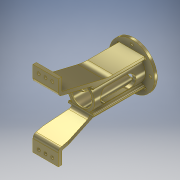
# Autodesk Inventor part: reverse gear standard 101
Saved by Autodesk Inventor 2017 (Build 210142000, 142)
## iProperties
Created: 2018-11-13
Part Number: reverse gear standard 101
Material: Generic
Document SubType Name: Modeling
Designer: User
Density: 1 g/cm^3
Appearance: Default
Author: User
Autodesk Inventor part; units mm, degrees
sketch "Sketch1" plane through (0, 0, 0) normal (0, 1, 0) x (-1, 0, 0)
  circle A0 centre (0, 0) radius 27
  circle A1 centre (0, 0) radius 14
  circle A2 centre (0, 0) radius 16
  circle A3 centre (0, 0) radius 12
  circle A4 centre (0, 0) radius 22 construction
  circle A5 centre (0, -22) radius 1.75
  circle A6 centre (15.5563, -15.5563) radius 1.75
  circle A7 centre (22, 0) radius 1.75
  circle A8 centre (15.5563, 15.5563) radius 1.75
  circle A9 centre (0, 22) radius 1.75
  circle A10 centre (-15.5563, 15.5563) radius 1.75
  circle A11 centre (-22, 0) radius 1.75
  circle A12 centre (-15.5563, -15.5563) radius 1.75
  dimension "d6" = 44
  dimension "d2" = 54
  dimension "d3" = 28
  dimension "d4" = 32
  dimension "d5" = 24
  dimension "d7" = 3.5
  dimension "d8" = 360
  dimension "d9" = 15.5564
  constraints: 12 centre point, 5 coincident, 1 vertical alignment, 19 other
  measures "d2" diameter of A0
  measures "d3" diameter of A1
  measures "d4" diameter of A2
  measures "d5" diameter of A3
  measures "d7" diameter of A5
  measures "d9" horizontal distance of A0.centre A6.centre
extrude "Extrusion1" add sketch "Sketch1" along normal blind 3 contours A0
extrude "Extrusion3" add sketch "Sketch1" against normal blind 60 contours A1 | A2
extrude "Extrusion4" cut sketch "Sketch1" against normal blind 1 contours A1
ref_plane "Work Plane1" through (0, 0, 0) normal (0, 0, 1) x (1, 0, 0)
ref_plane "Work Plane2" through (0, 0, 0) normal (1, 0, 0) x (0, 1, 0)
sketch "Sketch4" plane through (0, 0, 0) normal (1, 0, 0) x (0, 1, 0)
  line L0 (-102, -45) -> (-102, -30.9493)
  line L1 (-98.1581, -26.0853) -> (-63.8419, -17.9147)
  line L2 (-60, -12) -> (-60, 12)
  line L3 (-60, -13.0507) -> (-60, -12)
  line L4 (0, 27) -> (0, -27)
  line L5 (-60, -12) -> (0, -12)
  line L6 (-1, -12) -> (-60, -12)
  line L7 (0, -12) -> (0, -17)
  line L8 (0, -17) -> (-37.1036, -17)
  line L9 (-96.4652, -29.788) -> (-48.7347, -18.3716)
  line L10 (-102, -45) -> (-98, -45)
  line L11 (-98, -45) -> (-98, -31.7331)
  arc A0 (-96.4652, -29.788) -> (-98, -31.7331) centre (-96, -31.7331) ccw
  arc A1 (-98.1581, -26.0853) -> (-102, -30.9493) centre (-97, -30.9493) ccw
  arc A2 (-63.8419, -17.9147) -> (-60, -13.0507) centre (-65, -13.0507) ccw
  arc A3 (-37.1036, -17) -> (-48.7347, -18.3716) centre (-37.1036, -67) ccw
  point P0 (0, 0)
  point P1 (0, 0)
  point P2 (-102, -27)
  point P3 (0, 27)
  point P4 (0, -27)
  point P5 (-43, -17)
  point P6 (-3, -16)
  point P7 (-60, -16)
  dimension "d20" = 18
  dimension "d21" = 43
  dimension "d22" = 4
  dimension "d23" = 2
  dimension "d24" = 5
  dimension "d25" = 50
  dimension "d26" = 13.451
  dimension "d27" = 166.608
  dimension "d28" = 33
  dimension "d29" = 5
  dimension "d30" = 38
  constraints: 22 end point, 8 point on circle, 8 tangent, 5 point on line, 4 centre point, 2 perpendicular, 2 vertical, 1 equal radius, 1 horizontal, 5 other
  measures "d20" distance of L0.start point (-102, -27)
  measures "d21" distance of L7.end point (-43, -17)
  measures "d22" distance of L0.start L10.end
  measures "d23" radius of A0
  measures "d24" radius of A1
  measures "d25" radius of A3
  measures "d26" angle of L6 L9
  measures "d27" angle of L6 L1
  measures "d28" distance between parallel lines of L6 L10
  measures "d29" distance between parallel lines of L6 L8
  measures "d30" distance between parallel lines of L2 L11
extrude "Extrusion5" add sketch "Sketch4" along normal mid plane 30
ref_plane "Work Plane8" through (0, 0, -55) normal (0, 0, 1) x (1, 0, 0)
sketch "Sketch9" plane through (0, 0, -55) normal (0, 0, 1) x (1, 0, 0)
  line L0 (-15, 0) -> (-14.5672, 0) projected
  line L1 (14.5672, 0) -> (-14.5672, 0) projected
  line L2 (14.5672, 0) -> (15, 0) projected
  line L3 (15, -37.1036) -> (15, 0) projected
  line L4 (-15, -37.1036) -> (15, -37.1036) projected
  line L5 (-15, 0) -> (-15, -37.1036) projected
  line L6 (-15, -48.7347) -> (15, -48.7347) projected
  line L7 (15, -96.4652) -> (15, -48.7347) projected
  line L8 (-15, -96.4652) -> (15, -96.4652) projected
  line L9 (-15, -48.7347) -> (-15, -96.4652) projected
  line L10 (-15, -48.7347) -> (-15, -37.1036) projected
  line L11 (15, -37.1036) -> (15, -48.7347) projected
  line L12 (15, 0) -> (15, -60) projected
  line L13 (12, -1) -> (-12, -1) projected
  line L14 (14.5672, 0) -> (15, 0) projected
  line L15 (15, 0) -> (8, 0)
  line L16 (-14, 0) -> (14, 0) projected
  line L17 (-15, 0) -> (-15, -37.1036) projected
  line L18 (-15, 0) -> (-8, 0)
  line L19 (15, 0) -> (15, -89.9)
  line L20 (-15, 0) -> (-15, -89.9)
  line L21 (8, 0) -> (8, -44.2)
  line L22 (-8, 0) -> (-8, -44.2)
  line L23 (8, -44.2) -> (15, -89.9)
  line L24 (-8, -44.2) -> (-15, -89.9)
  point P0 (0, 0)
  point P1 (0, -1)
  point P2 (7.2111, 0)
  point P3 (-7.2111, 0)
  dimension "d85" = 7
  dimension "d86" = 7
  dimension "d87" = 89.9
  dimension "d88" = 89.9
  dimension "d89" = 44.2
  dimension "d90" = 44.2
  constraints: 16 end point, 4 point on line, 2 vertical
  measures "d85" distance of L2.end L15.end
  measures "d86" distance of L0.start L18.end
  measures "d87" distance of L2.end L19.end
  measures "d88" distance of L0.start L20.end
  measures "d89" distance of L15.end L21.end
  measures "d90" distance of L18.end L22.end
extrude "Extrusion7" cut sketch "Sketch9" along normal blind 40 contours L0 L1 L22 L4 L5 | L4 L22 L24 L6 L10 | L6 L24 L9 | L21 L1 L2 L3 L4 | L4 L11 L6 L23 L21 | L6 L7 L23
sketch "Sketch10" plane through (-15, -98, -31.7331) normal (0, 1, 0) x (1, 0, 0)
  line L0 (30, 13.2669) -> (0, 13.2669)
  circle A0 centre (7, 7.2669) radius 1.75
  circle A1 centre (15, 7.2669) radius 1.75
  circle A2 centre (23, 7.2669) radius 1.75
  point P0 (15, -31.7331)
  point P1 (15, -31.7331)
  dimension "d95" = 3.5
  dimension "d96" = 3.5
  dimension "d97" = 6
  dimension "d98" = 6
  dimension "d99" = 6
  dimension "d100" = 9.2195
  dimension "d101" = 16.1555
  dimension "d102" = 23.7697
  dimension "d103" = 45
  dimension "d104" = 45
  dimension "d105" = 47.4342
  dimension "d106" = 0
  dimension "d107" = 47.4342
  constraints: 3 centre point, 2 end point, 1 equal radius, 1 horizontal
  measures "d95" diameter of A0
  measures "d96" diameter of A1
  measures "d97" distance from line of A2.centre L0
  measures "d98" distance from line of A1.centre L0
  measures "d99" distance from line of A0.centre L0
  measures "d100" distance of L0.start A2.centre
  measures "d101" distance of L0.start A1.centre
  measures "d102" distance of L0.start A0.centre
  measures "d103" distance from line of point (15, -31.733) L0
  measures "d104" distance from line of point (15, -31.733) L0
  measures "d105" distance of point (15, -31.733) L0.start
  measures "d106" distance of point (15, -31.733) point (15, -31.733)
  measures "d107" distance of point (15, -31.733) L0.end
extrude "Extrusion8" cut sketch "Sketch10" against normal through all
mirror "Mirror1" about plane through (0, 0, 0) normal (0, 0, 1) of "Extrusion5"
mirror "Mirror2" about plane through (0, 0, 0) normal (0, 0, 1) of "Extrusion8"
fillet "Fillet1" radius 1 1 edges at (12, -60, 0)
ref_plane "Work Plane9" through (34, 0, 0) normal (1, 0, 0) x (0, 1, 0)
sketch "Sketch12" plane through (34, 0, 0) normal (1, 0, 0) x (0, 1, 0)
  arc A0 (-45, 8) -> (-45, -8) centre (-45, 0) ccw
  line L0 (-45, -8) -> (-19, -8)
  arc A1 (-19, -8) -> (-19, 8) centre (-19, 0) ccw
  line L1 (-19, 8) -> (-45, 8)
  point P0 (0, 0)
  point P1 (0, 0)
  dimension "d113" = 16
  dimension "d114" = 26
  dimension "d115" = 8
  dimension "d116" = 8
  dimension "d117" = 0
  dimension "d118" = 20.6155
  constraints: 4 end point, 4 point on circle, 4 tangent, 2 centre point, 2 horizontal
  measures "d113" diameter of A0
  measures "d114" distance of L0.start L0.end
  measures "d115" distance from line of point (0, 0) L1
  measures "d116" distance from line of point (0, 0) L1
  measures "d117" distance of point (0, 0) point (0, 0)
  measures "d118" distance of point (0, 0) L1.start
extrude "Extrusion9" cut sketch "Sketch12" against normal through all
fillet "Fillet2" radius 2 4 edges at (-15, -30, 12) (-15, -30, -12) (15, -30, -12) (15, -30, 12)
body "Solid1"
